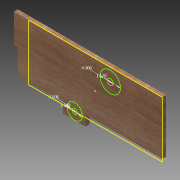
# Autodesk Inventor part: Robot Shooter Support Wall
Saved by Autodesk Inventor 2014 (Build 180170000, 170)
## iProperties
Created: 2016-01-28
Part Number: Robot Shooter Support Wall
Material: Wood (Birch)
Document SubType Name: Modeling
Designer: glasera
Density: 0.55 g/cm^3
Appearance: Birch - Natural Polished
Author: glasera
Autodesk Inventor part; units mm, degrees
ref_plane "YZ Plane" through (0, 0, 0) normal (1, 0, 0) x (0, 1, 0)
ref_plane "XZ Plane" through (0, 0, 0) normal (0, 1, 0) x (-1, 0, 0)
ref_plane "XY Plane" through (0, 0, 0) normal (0, 0, 1) x (1, 0, 0)
sketch "Sketch1" plane through (0, 0, 0) normal (0, 1, 0) x (-1, 0, 0)
  line L0 (332.74, 139.7) -> (-332.74, 139.7)
  line L1 (-332.74, 139.7) -> (-332.74, -139.7)
  line L2 (-332.74, -139.7) -> (332.74, -139.7)
  line L3 (332.74, -139.7) -> (332.74, 139.7)
  line L4 (332.74, 139.7) -> (-332.74, -139.7) construction
  line L5 (-332.74, 139.7) -> (332.74, -139.7) construction
  point P0 (0, 0)
  dimension "d0" = 665.48
  dimension "d1" = 279.4
  constraints: 12 end point, 2 midpoint, 2 parallel, 1 horizontal, 1 perpendicular
  measures "d0" distance of L2.end L1.end
  measures "d1" distance of L1.end L0.end
extrude "Extrusion1" add sketch "Sketch1" along normal blind 19.05
sketch "Sketch2" plane through (0, 19.05, 0) normal (0, 1, 0) x (1, 0, 0)
  circle A0 centre (73.2058, 76.2) radius 50.8
  circle A1 centre (-104.14, -139.7) radius 38.1
  line L0 (-332.74, -139.7) -> (332.74, -139.7) projected
  line L1 (332.74, -139.7) -> (332.74, 139.7) projected
  line L2 (332.74, 139.7) -> (-332.74, 139.7) projected
  line L3 (-332.74, 139.7) -> (-332.74, -139.7) projected
  circle A2 centre (-104.14, -139.7) radius 12.7
  circle A3 centre (73.2058, 76.2) radius 14.859
  point P0 (0, 0)
  dimension "d12" = 101.6
  dimension "d13" = 76.2
  dimension "d27" = 25.4
  dimension "d28" = 29.718
  constraints: 4 centre point, 2 coincident
  measures "d12" diameter of A0
  measures "d13" diameter of A1
  measures "d27" diameter of A2
  measures "d28" diameter of A3
sketch "Sketch4" plane through (-332.74, 0, 139.7) normal (0, 0, 1) x (1, 0, 0)
  line L0 (0, 0) -> (665.48, 0) projected
  line L1 (665.48, 0) -> (665.48, 19.05) projected
  line L2 (0, 19.05) -> (665.48, 19.05) projected
  line L3 (0, 0) -> (0, 19.05) projected
  point P0 (332.74, 0)
extrude "Extrusion3" add sketch "Sketch4" along normal blind 38.1
sketch "Sketch5" plane through (0, 19.05, 0) normal (0, 1, 0) x (1, 0, 0)
  line L0 (-332.74, -177.8) -> (-161.29, -177.8)
  line L1 (-161.29, -177.8) -> (-161.29, -127)
  line L2 (-161.29, -127) -> (-332.74, -127)
  line L3 (-332.74, -127) -> (-332.74, -177.8)
  line L4 (332.74, -177.8) -> (-48.2601, -177.8)
  line L5 (-48.2601, -177.8) -> (-48.2601, -127)
  line L6 (-48.2601, -127) -> (332.74, -127)
  line L7 (332.74, -127) -> (332.74, -177.8)
  line L8 (332.74, -177.8) -> (-48.2601, -177.8)
  line L9 (-48.2601, -177.8) -> (-48.2601, -127)
  line L10 (-48.2601, -127) -> (332.74, -127)
  line L11 (332.74, -127) -> (332.74, -177.8)
  point P0 (0, 0)
  dimension "d18" = 171.45
  dimension "d19" = 50.8
  constraints: 24 end point, 6 parallel, 3 horizontal, 3 perpendicular
  measures "d18" distance of L1.end L2.end
  measures "d19" distance of L0.end L1.end
extrude "Extrusion5" cut sketch "Sketch5" against normal blind 50.8
sketch "Sketch6" plane through (-332.74, 0, -139.7) normal (-1, 0, 0) x (0, 0, 1)
  line L0 (266.7, 0) -> (266.7, 19.05) projected
  line L1 (0, 19.05) -> (266.7, 19.05) projected
  line L2 (0, 0) -> (0, 19.05) projected
  line L3 (0, 0) -> (266.7, 0) projected
  point P0 (139.7, 0)
extrude "Extrusion6" add sketch "Sketch6" along normal blind 53.975
sketch "Sketch7" plane through (-386.715, 0, -139.7) normal (-1, 0, 0) x (0, 0, 1)
  line L0 (266.7, 19.05) -> (0, 19.05) projected
  line L1 (266.7, 19.05) -> (147.066, 19.05)
  line L2 (0, 0) -> (147.066, 0)
  line L3 (147.066, 0) -> (147.066, 19.05)
  line L4 (147.066, 19.05) -> (0, 19.05)
  line L5 (0, 19.05) -> (0, 0)
  point P0 (139.7, 0)
  dimension "d24" = 119.634
  constraints: 10 end point, 2 parallel, 1 horizontal, 1 perpendicular, 1 point on line
  measures "d24" distance of L0.start L1.end
extrude "Extrusion7" add sketch "Sketch7" along normal blind 19.05
body "Solid1"
